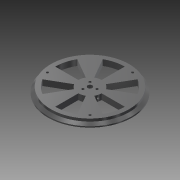
# Autodesk Inventor part: wheel
Saved by Autodesk Inventor 2011 (Build 150239000, 239)
## iProperties
Created: 2010-04-18
Part Number: wheel
Document SubType Name: Modeling
Designer: lucio
Density: 0.94 g/cm^3
Material: UHMW, Black
Mass: 93.0991 g
Surface Area: 347.259 cm^2
Volume: 99.0416 cm^3
GlobalPropertyList: <PropertyList/>
Author: lucio
Autodesk Inventor part; units mm, degrees
ref_plane "YZ Plane" through (0, 0, 0) normal (1, 0, 0) x (0, 1, 0)
ref_plane "XZ Plane" through (0, 0, 0) normal (0, 1, 0) x (-1, 0, 0)
sketch "Sketch1" plane through (0, 0, 0) normal (0, 0, 1) x (1, 0, 0)
  circle A0 centre (0, 0) radius 72.5
  circle A1 centre (0, 0) radius 67.5
  circle A2 centre (0, 0) radius 4
  line L0 (0, 20) -> (0, 60)
  arc A3 (0, 20) -> (-10, 17.3205) centre (0, 0) ccw
  line L1 (0, 0) -> (-10, 17.3205) construction
  line L2 (0, 0) -> (0, 20) construction
  arc A4 (0, 60) -> (-30, 51.9615) centre (0, 0) ccw
  line L3 (0, 0) -> (-30, 51.9615) construction
  line L4 (0, 0) -> (0, 60) construction
  line L5 (-10, 17.3205) -> (-30, 51.9615)
  line L6 (-17.3205, 10) -> (-51.9615, 30)
  arc A5 (-17.3205, 10) -> (-20, 0) centre (0, 0) ccw
  line L7 (0, 0) -> (-20, 0) construction
  line L8 (0, 0) -> (-17.3205, 10) construction
  arc A6 (-51.9615, 30) -> (-60, 0) centre (0, 0) ccw
  line L9 (0, 0) -> (-60, 0) construction
  line L10 (0, 0) -> (-51.9615, 30) construction
  line L11 (-20, 0) -> (-60, 0)
  line L12 (-17.3205, -10) -> (-51.9615, -30)
  arc A7 (-17.3205, -10) -> (-10, -17.3205) centre (0, 0) ccw
  line L13 (0, 0) -> (-10, -17.3205) construction
  line L14 (0, 0) -> (-17.3205, -10) construction
  arc A8 (-51.9615, -30) -> (-30, -51.9615) centre (0, 0) ccw
  line L15 (0, 0) -> (-30, -51.9615) construction
  line L16 (0, 0) -> (-51.9615, -30) construction
  line L17 (-10, -17.3205) -> (-30, -51.9615)
  line L18 (0, -20) -> (0, -60)
  arc A9 (0, -20) -> (10, -17.3205) centre (0, 0) ccw
  line L19 (0, 0) -> (10, -17.3205) construction
  line L20 (0, 0) -> (0, -20) construction
  arc A10 (0, -60) -> (30, -51.9615) centre (0, 0) ccw
  line L21 (0, 0) -> (30, -51.9615) construction
  line L22 (0, 0) -> (0, -60) construction
  line L23 (10, -17.3205) -> (30, -51.9615)
  line L24 (17.3205, -10) -> (51.9615, -30)
  arc A11 (17.3205, -10) -> (20, 0) centre (0, 0) ccw
  line L25 (0, 0) -> (20, 0) construction
  line L26 (0, 0) -> (17.3205, -10) construction
  arc A12 (51.9615, -30) -> (60, 0) centre (0, 0) ccw
  line L27 (0, 0) -> (60, 0) construction
  line L28 (0, 0) -> (51.9615, -30) construction
  line L29 (20, 0) -> (60, 0)
  line L30 (17.3205, 10) -> (51.9615, 30)
  arc A13 (17.3205, 10) -> (10, 17.3205) centre (0, 0) ccw
  line L31 (0, 0) -> (10, 17.3205) construction
  line L32 (0, 0) -> (17.3205, 10) construction
  arc A14 (51.9615, 30) -> (30, 51.9615) centre (0, 0) ccw
  line L33 (0, 0) -> (30, 51.9615) construction
  line L34 (0, 0) -> (51.9615, 30) construction
  line L35 (10, 17.3205) -> (30, 51.9615)
  point P0 (0, 10)
  point P1 (-2.5882, 9.6593)
  point P2 (-5, 8.6603)
  point P3 (-7.0711, 7.0711)
  point P4 (-8.6603, 5)
  point P5 (-9.6593, 2.5882)
  point P6 (-10, 0)
  point P7 (-9.6593, -2.5882)
  point P8 (-8.6603, -5)
  point P9 (-7.0711, -7.0711)
  point P10 (-5, -8.6603)
  point P11 (-2.5882, -9.6593)
  point P12 (0, -10)
  point P13 (2.5882, -9.6593)
  point P14 (5, -8.6603)
  point P15 (7.0711, -7.0711)
  point P16 (8.6603, -5)
  point P17 (9.6593, -2.5882)
  point P18 (10, 0)
  point P19 (9.6593, 2.5882)
  point P20 (8.6603, 5)
  point P21 (7.0711, 7.0711)
  point P22 (5, 8.6603)
  point P23 (2.5882, 9.6593)
  point P24 (15.5291, -57.9555)
  point P25 (30, -51.9615)
  point P26 (42.4264, -42.4264)
  point P27 (51.9615, -30)
  point P28 (57.9555, -15.5291)
  point P29 (60, 0)
  point P30 (57.9555, 15.5291)
  point P31 (51.9615, 30)
  point P32 (42.4264, 42.4264)
  point P33 (30, 51.9615)
  point P34 (15.5291, 57.9555)
  point P35 (0, 60)
  point P36 (-15.5291, 57.9555)
  point P37 (-30, 51.9615)
  point P38 (-42.4264, 42.4264)
  point P39 (-51.9615, 30)
  point P40 (-57.9555, 15.5291)
  point P41 (-60, 0)
  point P42 (-57.9555, -15.5291)
  point P43 (-51.9615, -30)
  point P44 (-42.4264, -42.4264)
  point P45 (-30, -51.9615)
  point P46 (-15.5291, -57.9555)
  dimension "d1" = 135
  dimension "d2" = 8
  dimension "d11" = 40
  dimension "d12" = 20
  dimension "d13" = 30
  dimension "d14" = 30
  dimension "d17" = 360
  dimension "d34" = 10
  dimension "d37" = 360
  dimension "d48" = 360
  dimension "d57" = 145
  constraints: 72 end point, 24 point on circle, 15 centre point, 13 coincident, 1 collinear, 1 point on line, 1 vertical, 133 other
  measures "d1" diameter of A1
  measures "d2" diameter of A2
  measures "d11" distance of L0.start L0.end
  measures "d12" distance of point (0, 0) L0.start
  measures "d13" angle of L2 L1
  measures "d14" angle of L4 L3
  measures "d34" distance of point (0, 0) point (0, 10)
  measures "d57" diameter of A0
extrude "Extrusion1" add sketch "Sketch1" along normal blind 10 contours A1
extrude "Extrusion2" add sketch "Sketch1" along normal blind 5.5 contours A0
hole "Hole2" at (-2.5882, -9.6593, 0) at (-7.0711, 7.0711, 0) at (9.6593, 2.5882, 0) direction (0, 0, 1) diameter 4 end through all counterbore diameter 7 counterbore depth 4
hole "Hole3" at (42.4264, -42.4264, 0) at (-57.9555, -15.5291, 0) at (15.5291, 57.9555, 0) direction (0, 0, 1) diameter 4 end through all counterbore diameter 7 counterbore depth 4
chamfer "Chamfer2" distance 3.5 distance2 5 1 edges at (-72.5, 0, 5.5) measured on face at (72.06, -7.9756, 1.8333)
ref_plane "Work Plane3" through (19.3185, -5.1764, 0) normal (-0.9659, 0.2588, 0) x (-0.2588, -0.9659, 0)
sketch "Sketch3" plane through (19.3185, -5.1764, 0) normal (-0.9659, 0.2588, 0) x (-0.2588, -0.9659, 0)
  point P0 (0, 0)
  point P1 (0, 5)
  dimension "d61" = 5
  measures "d61" distance of point (0, 0) point (0, 5)
hole "Hole4" at (19.3185, -5.1764, 5) direction (-0.9659, 0.2588, 0) diameter 3.5 depth 20
body "Solid1"
